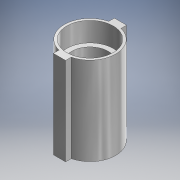
# Autodesk Inventor part: AA042
Saved by Autodesk Inventor 2017 SP1 (Build 210196100, 196)
## iProperties
Created: 2018-01-24
Part Number: AA042
Material: ABS Plastic
Document SubType Name: Modeling
Designer: Zach
Density: 1.06 g/cm^3
Appearance: CR White
Author: Zach
Autodesk Inventor part; units mm, degrees
ref_plane "YZ Plane" through (0, 0, 0) normal (1, 0, 0) x (0, 1, 0)
ref_plane "XZ Plane" through (0, 0, 0) normal (0, 1, 0) x (-1, 0, 0)
ref_plane "XY Plane" through (0, 0, 0) normal (0, 0, 1) x (1, 0, 0)
sketch "Sketch1" plane through (0, 0, 0) normal (0, 0, 1) x (1, 0, 0)
  circle A0 centre (0, 0) radius 3.75
  line L0 (1.25, -6.25) -> (-1.25, -6.25)
  line L1 (-1.25, -6.25) -> (-1.25, 6.25) construction
  line L2 (-1.25, 6.25) -> (1.25, 6.25)
  line L3 (1.25, 6.25) -> (1.25, -6.25) construction
  circle A1 centre (0, 0) radius 5.25
  line L4 (1.25, -5.099) -> (1.25, -6.25)
  line L5 (-1.25, -6.25) -> (-1.25, -5.099)
  line L6 (-1.25, 6.25) -> (-1.25, 5.099)
  line L7 (1.25, 6.25) -> (1.25, 5.099)
  arc A2 (-1.25, -5.099) -> (1.25, -5.099) centre (0, 0) ccw
  arc A3 (1.25, 5.099) -> (-1.25, 5.099) centre (0, 0) ccw
  point P0 (0, 6.25)
  point P1 (1.25, 0)
  dimension "d1" = 7.5
  dimension "d10" = 2.5
  dimension "d11" = 12.5
  dimension "d12" = 10.5
  constraints: 16 end point, 8 point on circle, 4 centre point, 4 point on line, 3 coincident, 2 concentric, 2 midpoint, 2 parallel, 1 collinear, 1 horizontal, 1 horizontal alignment, 1 perpendicular, 1 vertical alignment
  measures "d1" diameter of A0
  measures "d10" distance of L1.end L2.end
  measures "d11" distance of L2.end L0.start
  measures "d12" diameter of A1
extrude "Extrusion1" add sketch "Sketch1" along normal blind 12
sketch "Sketch5" plane through (0, 0, 0) normal (0, 0, -1) x (-1, 0, 0)
  circle A0 centre (0, 0) radius 3.75 projected
  circle A1 centre (0, 0) radius 3.75 projected
  line L0 (-1.25, -6.25) -> (-1.25, -5.099) projected
  line L1 (1.25, -6.25) -> (-1.25, -6.25) projected
  line L2 (1.25, -5.099) -> (1.25, -6.25) projected
  arc A2 (1.25, -5.099) -> (1.25, 5.099) centre (0, 0) ccw projected
  line L3 (1.25, 6.25) -> (1.25, 5.099) projected
  line L4 (-1.25, 6.25) -> (1.25, 6.25) projected
  line L5 (-1.25, 5.099) -> (-1.25, 6.25) projected
  arc A3 (-1.25, 5.099) -> (-1.25, -5.099) centre (0, 0) ccw projected
  circle A4 centre (0, 0) radius 1.5
  dimension "d13" = 3
  constraints: 1 centre point, 1 coincident
  measures "d13" diameter of A4
extrude "Extrusion4" add sketch "Sketch5" along normal blind 2 contours A0 | L0 A3 L5 L4 L3 A2 L2 L1
sketch "Sketch6" plane through (0, 0, 0) normal (0, 0, 1) x (1, 0, 0)
  line L0 (0.625, 6.25) -> (-0.625, 6.25)
  line L1 (-0.625, 6.25) -> (-0.625, -6.25) construction
  line L2 (-0.625, -6.25) -> (0.625, -6.25)
  line L3 (0.625, -6.25) -> (0.625, 6.25) construction
  line L4 (-1.25, 6.25) -> (1.25, 6.25) projected
  circle A0 centre (0, 0) radius 1.5 construction
  arc A1 (0.625, 1.3636) -> (-0.625, 1.3636) centre (0, 0) ccw
  arc A2 (-0.625, -1.3636) -> (0.625, -1.3636) centre (0, 0) ccw
  line L5 (0.625, 6.25) -> (0.625, 1.3636)
  line L6 (-0.625, 6.25) -> (-0.625, 1.3636)
  line L7 (0.625, -1.3636) -> (0.625, -6.25)
  line L8 (-0.625, -1.3636) -> (-0.625, -6.25)
  point P0 (0, 0)
  point P1 (0, 6.25)
  point P2 (0.625, 0)
  dimension "d16" = 1.25
  constraints: 16 end point, 8 point on circle, 5 point on line, 3 parallel, 2 centre point, 2 collinear, 2 concentric, 2 midpoint, 1 horizontal, 1 horizontal alignment, 1 perpendicular, 1 vertical, 1 vertical alignment
  measures "d16" distance of L1.end L2.end
extrude "Extrusion5" add sketch "Sketch6" along normal blind 2
sketch "Sketch9" plane through (0, 0, 12) normal (0, 0, 1) x (1, 0, 0)
  circle A0 centre (0, 0) radius 3.75 construction
  line L0 (1.25, -6.25) -> (1.25, -5.099) projected
  arc A1 (1.25, -5.099) -> (1.25, 5.099) centre (0, 0) ccw projected
  line L1 (1.25, 5.099) -> (1.25, 6.25) projected
  line L2 (1.25, 6.25) -> (-1.25, 6.25) projected
  line L3 (-1.25, 6.25) -> (-1.25, 5.099) projected
  arc A2 (-1.25, 5.099) -> (-1.25, -5.099) centre (0, 0) ccw projected
  line L4 (-1.25, -5.099) -> (-1.25, -6.25) projected
  line L5 (-1.25, -6.25) -> (1.25, -6.25) projected
  circle A3 centre (0, 0) radius 4.75
  dimension "d23" = 9.5
  constraints: 1 centre point, 1 coincident
  measures "d23" diameter of A3
extrude "Extrusion7" add sketch "Sketch9" along normal blind 4
body "Solid1"
